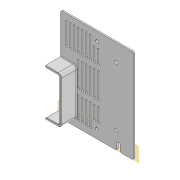
# Autodesk Inventor part: fechamento2
Saved by Autodesk Inventor 2020 (Build 240168000, 168)
## iProperties
Created: 2022-08-02
Part Number: fechamento2
Material: Genérico
Document SubType Name: Modeling
Designer: gabri
Density: 1 g/cm^3
Appearance: Padrão
Author: gabri
Autodesk Inventor part; units mm, degrees
ref_plane "YZ Plane" through (0, 0, 0) normal (1, 0, 0) x (0, 1, 0)
ref_plane "XZ Plane" through (0, 0, 0) normal (0, 1, 0) x (-1, 0, 0)
ref_plane "XY Plane" through (0, 0, 0) normal (0, 0, 1) x (1, 0, 0)
ref_plane "Plano de trabalho1" through (0, 0, 0) normal (0, 0, 1) x (1, 0, 0)
sketch "Esboço1" plane through (0, 0, 0) normal (0, 0, 1) x (1, 0, 0)
  arc A0 (62, 11) -> (61, 12) centre (61, 11) ccw projected
  line L0 (61, 12) -> (49, 12) projected
  arc A1 (49, 12) -> (48, 11) centre (49, 11) ccw projected
  line L1 (48, 1) -> (48, 11) projected
  arc A2 (47, 0) -> (48, 1) centre (47, 1) ccw projected
  line L2 (11, 0) -> (47, 0) projected
  arc A3 (10, 1) -> (11, 0) centre (11, 1) ccw projected
  line L3 (10, 1) -> (10, 9) projected
  line L4 (0, 9) -> (10, 9) projected
  line L5 (0, -8) -> (0, 9) projected
  line L6 (0, -8) -> (110, -8) projected
  line L7 (110, -8) -> (110, 9) projected
  line L8 (100, 9) -> (110, 9) projected
  line L9 (100, 1) -> (100, 9) projected
  arc A4 (99, 0) -> (100, 1) centre (99, 1) ccw projected
  line L10 (63, 0) -> (99, 0) projected
  arc A5 (62, 1) -> (63, 0) centre (63, 1) ccw projected
  line L11 (62, 11) -> (62, 1) projected
  circle A6 centre (55, 6) radius 2.25 projected
  arc A7 (48, 96) -> (49, 95) centre (49, 96) ccw projected
  line L12 (61, 95) -> (49, 95) projected
  arc A8 (61, 95) -> (62, 96) centre (61, 96) ccw projected
  line L13 (62, 106) -> (62, 96) projected
  arc A9 (63, 107) -> (62, 106) centre (63, 106) ccw projected
  line L14 (63, 107) -> (99.2679, 107) projected
  spline S0 degree 3 poles (101, 106) (100.7229, 106.2771) (100.3848, 106.6039) (99.8153, 106.9104) (99.5228, 107) (99.2679, 107) knots 0 0 0 0 0.117563 0.117563 0.194026 0.194026 0.194026 0.194026 projected
  line L15 (101, 98) -> (101, 106) projected
  line L16 (110, 98) -> (101, 98) projected
  line L17 (110, 115) -> (110, 98) projected
  line L18 (0, 115) -> (110, 115) projected
  line L19 (0, 115) -> (0, 98) projected
  line L20 (10, 98) -> (0, 98) projected
  line L21 (10, 106) -> (10, 98) projected
  arc A10 (11, 107) -> (10, 106) centre (11, 106) ccw projected
  line L22 (11, 107) -> (47, 107) projected
  arc A11 (48, 106) -> (47, 107) centre (47, 106) ccw projected
  line L23 (48, 96) -> (48, 106) projected
  circle A12 centre (55, 101) radius 2.25 projected
  line L24 (109.5, 114) -> (0.5, 114)
  line L25 (0.5, 114) -> (0.5, -7)
  line L26 (0.5, -7) -> (109.5, -7)
  line L27 (109.5, -7) -> (109.5, 114)
  line L28 (55, 101.5) -> (55, 100.5)
  line L29 (55, 101.5) -> (55, 100.5) construction
  line L30 (52.75, 101.5) -> (52.75, 100.5)
  line L31 (57.25, 100.5) -> (57.25, 101.5)
  arc A13 (57.25, 101.5) -> (52.75, 101.5) centre (55, 101.5) ccw
  arc A14 (52.75, 100.5) -> (57.25, 100.5) centre (55, 100.5) ccw
  circle A15 centre (55, 6) radius 0.25
  line L32 (55, 6.25) -> (55, 5.75) construction
  line L33 (52.75, 6.25) -> (52.75, 5.75)
  line L34 (57.25, 5.75) -> (57.25, 6.25)
  arc A16 (57.25, 6.25) -> (52.75, 6.25) centre (55, 6.25) ccw
  arc A17 (52.75, 5.75) -> (57.25, 5.75) centre (55, 5.75) ccw
  circle A18 centre (86.5, 96) radius 5
  circle A19 centre (86.5, 65) radius 5
  line L35 (45.1388, 99) -> (45.1388, 67) construction
  line L36 (46.7388, 99) -> (46.7388, 67)
  line L37 (43.5388, 67) -> (43.5388, 99)
  arc A20 (46.7388, 99) -> (43.5388, 99) centre (45.1388, 99) ccw
  arc A21 (43.5388, 67) -> (46.7388, 67) centre (45.1388, 67) ccw
  line L38 (45.1388, 35) -> (45.1388, 3) construction
  line L39 (46.7388, 35) -> (46.7388, 3)
  line L40 (43.5388, 3) -> (43.5388, 35)
  arc A22 (46.7388, 35) -> (43.5388, 35) centre (45.1388, 35) ccw
  arc A23 (43.5388, 3) -> (46.7388, 3) centre (45.1388, 3) ccw
  arc A24 (37.5388, 67) -> (40.7388, 67) centre (39.1388, 67) ccw
  arc A25 (40.7388, 35) -> (37.5388, 35) centre (39.1388, 35) ccw
  line L41 (40.7388, 99) -> (40.7388, 67)
  line L42 (39.1388, 99) -> (39.1388, 67) construction
  line L43 (37.5388, 67) -> (37.5388, 99)
  arc A26 (40.7388, 99) -> (37.5388, 99) centre (39.1388, 99) ccw
  line L44 (40.7388, 35) -> (40.7388, 3)
  line L45 (39.1388, 35) -> (39.1388, 3) construction
  line L46 (37.5388, 3) -> (37.5388, 35)
  arc A27 (37.5388, 3) -> (40.7388, 3) centre (39.1388, 3) ccw
  arc A28 (31.5388, 67) -> (34.7388, 67) centre (33.1388, 67) ccw
  arc A29 (34.7388, 35) -> (31.5388, 35) centre (33.1388, 35) ccw
  line L47 (34.7388, 99) -> (34.7388, 67)
  line L48 (33.1388, 99) -> (33.1388, 67) construction
  line L49 (31.5388, 67) -> (31.5388, 99)
  arc A30 (34.7388, 99) -> (31.5388, 99) centre (33.1388, 99) ccw
  line L50 (34.7388, 35) -> (34.7388, 3)
  line L51 (33.1388, 35) -> (33.1388, 3) construction
  line L52 (31.5388, 3) -> (31.5388, 35)
  arc A31 (31.5388, 3) -> (34.7388, 3) centre (33.1388, 3) ccw
  arc A32 (25.5388, 67) -> (28.7388, 67) centre (27.1388, 67) ccw
  arc A33 (28.7388, 35) -> (25.5388, 35) centre (27.1388, 35) ccw
  line L53 (28.7388, 99) -> (28.7388, 67)
  line L54 (27.1388, 99) -> (27.1388, 67) construction
  line L55 (25.5388, 67) -> (25.5388, 99)
  arc A34 (28.7388, 99) -> (25.5388, 99) centre (27.1388, 99) ccw
  line L56 (28.7388, 35) -> (28.7388, 3)
  line L57 (27.1388, 35) -> (27.1388, 3) construction
  line L58 (25.5388, 3) -> (25.5388, 35)
  arc A35 (25.5388, 3) -> (28.7388, 3) centre (27.1388, 3) ccw
  arc A36 (19.5388, 67) -> (22.7388, 67) centre (21.1388, 67) ccw
  arc A37 (22.7388, 35) -> (19.5388, 35) centre (21.1388, 35) ccw
  line L59 (22.7388, 99) -> (22.7388, 67)
  line L60 (21.1388, 99) -> (21.1388, 67) construction
  line L61 (19.5388, 67) -> (19.5388, 99)
  arc A38 (22.7388, 99) -> (19.5388, 99) centre (21.1388, 99) ccw
  line L62 (22.7388, 35) -> (22.7388, 3)
  line L63 (21.1388, 35) -> (21.1388, 3) construction
  line L64 (19.5388, 3) -> (19.5388, 35)
  arc A39 (19.5388, 3) -> (22.7388, 3) centre (21.1388, 3) ccw
  arc A40 (13.5388, 67) -> (16.7388, 67) centre (15.1388, 67) ccw
  arc A41 (16.7388, 35) -> (13.5388, 35) centre (15.1388, 35) ccw
  line L65 (16.7388, 99) -> (16.7388, 67)
  line L66 (15.1388, 99) -> (15.1388, 67) construction
  line L67 (13.5388, 67) -> (13.5388, 99)
  arc A42 (16.7388, 99) -> (13.5388, 99) centre (15.1388, 99) ccw
  line L68 (16.7388, 35) -> (16.7388, 3)
  line L69 (15.1388, 35) -> (15.1388, 3) construction
  line L70 (13.5388, 3) -> (13.5388, 35)
  arc A43 (13.5388, 3) -> (16.7388, 3) centre (15.1388, 3) ccw
  arc A44 (7.5388, 67) -> (10.7388, 67) centre (9.1388, 67) ccw
  arc A45 (10.7388, 35) -> (7.5388, 35) centre (9.1388, 35) ccw
  line L71 (10.7388, 99) -> (10.7388, 67)
  line L72 (9.1388, 99) -> (9.1388, 67) construction
  line L73 (7.5388, 67) -> (7.5388, 99)
  arc A46 (10.7388, 99) -> (7.5388, 99) centre (9.1388, 99) ccw
  line L74 (10.7388, 35) -> (10.7388, 3)
  line L75 (9.1388, 35) -> (9.1388, 3) construction
  line L76 (7.5388, 3) -> (7.5388, 35)
  arc A47 (7.5388, 3) -> (10.7388, 3) centre (9.1388, 3) ccw
  line L77 (51.1388, 35) -> (51.1388, 15.5537) construction
  line L78 (49.5388, 35) -> (49.5388, 15.5537)
  line L79 (52.7388, 15.5537) -> (52.7388, 35)
  arc A48 (52.7388, 35) -> (49.5388, 35) centre (51.1388, 35) ccw
  arc A49 (49.5388, 15.5537) -> (52.7388, 15.5537) centre (51.1388, 15.5537) ccw
  line L80 (55.5388, 35) -> (55.5388, 15.5537)
  line L81 (57.1388, 35) -> (57.1388, 15.5537) construction
  arc A50 (55.5388, 15.5537) -> (58.7388, 15.5537) centre (57.1388, 15.5537) ccw
  line L82 (58.7388, 15.5537) -> (58.7388, 35)
  arc A51 (58.7388, 35) -> (55.5388, 35) centre (57.1388, 35) ccw
  line L83 (61.5388, 35) -> (61.5388, 15.5537)
  line L84 (63.1388, 35) -> (63.1388, 15.5537) construction
  arc A52 (61.5388, 15.5537) -> (64.7388, 15.5537) centre (63.1388, 15.5537) ccw
  line L85 (64.7388, 15.5537) -> (64.7388, 35)
  arc A53 (64.7388, 35) -> (61.5388, 35) centre (63.1388, 35) ccw
  line L86 (69.1388, 35) -> (69.1388, 3) construction
  line L87 (67.5388, 35) -> (67.5388, 3)
  line L88 (70.7388, 3) -> (70.7388, 35)
  arc A54 (70.7388, 35) -> (67.5388, 35) centre (69.1388, 35) ccw
  arc A55 (67.5388, 3) -> (70.7388, 3) centre (69.1388, 3) ccw
  arc A56 (76.7388, 35) -> (73.5388, 35) centre (75.1388, 35) ccw
  line L89 (73.5388, 35) -> (73.5388, 3)
  line L90 (75.1388, 35) -> (75.1388, 3) construction
  arc A57 (73.5388, 3) -> (76.7388, 3) centre (75.1388, 3) ccw
  line L91 (76.7388, 3) -> (76.7388, 35)
  arc A58 (82.7388, 35) -> (79.5388, 35) centre (81.1388, 35) ccw
  line L92 (79.5388, 35) -> (79.5388, 3)
  line L93 (81.1388, 35) -> (81.1388, 3) construction
  arc A59 (79.5388, 3) -> (82.7388, 3) centre (81.1388, 3) ccw
  line L94 (82.7388, 3) -> (82.7388, 35)
  arc A60 (88.7388, 35) -> (85.5388, 35) centre (87.1388, 35) ccw
  line L95 (85.5388, 35) -> (85.5388, 3)
  line L96 (87.1388, 35) -> (87.1388, 3) construction
  arc A61 (85.5388, 3) -> (88.7388, 3) centre (87.1388, 3) ccw
  line L97 (88.7388, 3) -> (88.7388, 35)
  arc A62 (94.7388, 35) -> (91.5388, 35) centre (93.1388, 35) ccw
  line L98 (91.5388, 35) -> (91.5388, 3)
  line L99 (93.1388, 35) -> (93.1388, 3) construction
  arc A63 (91.5388, 3) -> (94.7388, 3) centre (93.1388, 3) ccw
  line L100 (94.7388, 3) -> (94.7388, 35)
  line L101 (97.5388, 35) -> (97.5388, 3)
  line L102 (99.1388, 35) -> (99.1388, 3) construction
  line L103 (100.7388, 3) -> (100.7388, 35)
  arc A64 (100.7388, 35) -> (97.5388, 35) centre (99.1388, 35) ccw
  arc A65 (97.5388, 3) -> (100.7388, 3) centre (99.1388, 3) ccw
  point P0 (0, 0)
  point P1 (55, 101)
  point P2 (45.1388, 83)
  point P3 (45.1388, 19)
  point P4 (42, 106)
  point P5 (39.1388, 83)
  point P6 (39.1388, 19)
  point P7 (36, 106)
  point P8 (33.1388, 83)
  point P9 (33.1388, 19)
  point P10 (30, 106)
  point P11 (27.1388, 83)
  point P12 (27.1388, 19)
  point P13 (24, 106)
  point P14 (21.1388, 83)
  point P15 (21.1388, 19)
  point P16 (18, 106)
  point P17 (15.1388, 83)
  point P18 (15.1388, 19)
  point P19 (12, 106)
  point P20 (9.1388, 83)
  point P21 (9.1388, 19)
  point P22 (51.1388, 25.2768)
  point P23 (57.1388, 25.2768)
  point P24 (63.1388, 25.2768)
  point P25 (69.1388, 19)
  point P26 (75.1388, 19)
  point P27 (81.1388, 19)
  point P28 (87.1388, 19)
  point P29 (93.1388, 19)
  point P30 (99.1388, 19)
  point P31 (10, 100.3484)
  point P32 (7.5388, 98)
  dimension "d0" = 0.5
  dimension "d1" = 0.5
  dimension "d2" = 1
  dimension "d3" = 1
  dimension "d4" = 0.5
  dimension "d5" = 0.5
  dimension "d6" = 4.5
  dimension "d7" = 0.5
  dimension "d8" = 4.5
  dimension "d9" = 10
  dimension "d10" = 10
  dimension "d11" = 18
  dimension "d12" = 23
  dimension "d13" = 23
  dimension "d14" = 31
  dimension "d15" = 32
  dimension "d16" = 32
  dimension "d17" = 31
  dimension "d18" = 26
  dimension "d19" = 3.2
  dimension "d20" = 3.2
  dimension "d23" = 6
  dimension "d30" = 3.2
  dimension "d31" = 6
  dimension "d34" = 6
  dimension "d39" = 3.2
  dimension "d40" = 6
  dimension "d43" = 6
  dimension "d50" = 6
  dimension "d69" = 32
  dimension "d70" = 26
  dimension "d71" = 19.4463
  dimension "d72" = 32.2769
  constraints: 210 end point, 102 point on circle, 53 centre point, 24 tangent, 14 point on line, 9 equal length, 6 midpoint, 5 horizontal, 5 vertical, 1 coincident, 1 perpendicular, 234 other
  measures "d0" distance between parallel lines of L17 L27
  measures "d1" distance from line of L19.end L25
  measures "d2" distance between parallel lines of L18 L24
  measures "d3" distance between parallel lines of L6 L26
  measures "d4" distance of L28.start A12.centre
  measures "d5" distance of L28.end A12.centre
  measures "d6" diameter of A14
  measures "d7" diameter of A15
  measures "d8" diameter of A17
  measures "d9" diameter of A18
  measures "d10" diameter of A19
  measures "d11" distance from line of L24 A18.centre
  measures "d12" distance from line of L27 A18.centre
  measures "d13" distance from line of L27 A19.centre
  measures "d14" distance of A19.centre A18.centre
  measures "d15" distance of L35.start L35.end
  measures "d16" distance of L38.start L38.end
  measures "d17" distance from line of L24 point (45.139, 83)
  measures "d18" distance from line of L26 point (45.139, 19)
  measures "d19" distance between parallel lines of L37 L36
  measures "d20" distance between parallel lines of L40 L39
  measures "d23" distance of L23.end point (42, 106)
  measures "d30" diameter of A49
  measures "d31" distance between parallel lines of L40 L78
  measures "d34" distance of L77.start L81.start
  measures "d39" diameter of A55
  measures "d40" horizontal distance of point (63.139, 25.277) point (69.139, 19)
  measures "d43" distance of L86.start L90.start
  measures "d50" distance of L98.start L101.start
  measures "d69" distance of L103.start L103.end
  measures "d70" distance from line of L26 point (69.139, 19)
  measures "d71" distance of L85.start L85.end
  measures "d72" distance from line of L26 point (57.139, 25.277)
extrude "Extrusão1" add sketch "Esboço1" along normal blind 2 contours L11 A5 L10 A4 L9 A65 L103 L8 L27 L26 L25 L4 L76 A47 L3 A3 L2 A2 L1 A1 L0 A0 | A0 L0 A1 L1 A2 L2 A3 L3 A47 L74 A45 L76 L4 L25 L20 L73 A44 L71 A46 L21 A10 L22 A11 L23 A7 L12 A8 L13 A9 L14 S0 L15 L16 L27 L8 L103 A64 L101 A65 L9 A4 L10 A5 L11 | L16 L15 S0 L14 A9 L13 A8 L12 A7 L23 A11 L22 A10 L21 A46 L73 L20 L25 L24 L27 | L20 L21 A46 L71 A44 L73 | A19 | L36 A21 L37 A20 | L43 A26 L41 A24 | L49 A30 L47 A28 | L55 A34 L53 A32 | L61 A38 L59 A36 | L67 A42 L65 A40
fillet "Arredondamento2" radius 2 4 edges at (109.5, -7, 1) (0.5, -7, 1) (0.5, 114, 1) (109.5, 114, 1)
sketch "Esboço5" plane through (0, 0, 2) normal (0, 0, 1) x (1, 0, 0)
  line L0 (115.4408, 125.4617) -> (-12.5595, 125.4617)
  line L1 (-12.5595, 125.4617) -> (-12.5595, 63)
  line L2 (-12.5595, 63) -> (115.4408, 63)
  line L3 (115.4408, 63) -> (115.4408, 125.4617)
  line L4 (2.5, -7) -> (107.5, -7) projected
  point P0 (0, 0)
  dimension "d66" = 70
  constraints: 8 end point, 2 parallel, 1 horizontal, 1 perpendicular
  measures "d66" distance between parallel lines of L4 L2
extrude "Extrusão5" cut sketch "Esboço5" against normal blind 2.2
mirror "Espelhamento1" about plane through (115.4408, 63, 2) normal (0, 1, 0)
sketch "Esboço6" plane through (0, 0, 2) normal (0, 0, 1) x (1, 0, 0)
  line L0 (0.5, 131) -> (0.5, -5) projected
  line L1 (0.5, 63) -> (46.0074, 63)
  arc A0 (7.5388, 91) -> (10.7388, 91) centre (9.1388, 91) ccw projected
  line L2 (9.1388, 89.4) -> (9.1388, 36.6)
  arc A1 (10.7388, 35) -> (7.5388, 35) centre (9.1388, 35) ccw projected
  line L3 (9.1388, 44.7338) -> (9.1388, 81.2662) construction
  line L4 (10.7388, 44.7338) -> (10.7388, 81.2662)
  line L5 (7.5388, 81.2662) -> (7.5388, 44.7338)
  arc A2 (7.5388, 44.7338) -> (10.7388, 44.7338) centre (9.1388, 44.7338) ccw
  arc A3 (10.7388, 81.2662) -> (7.5388, 81.2662) centre (9.1388, 81.2662) ccw
  line L6 (15.1388, 44.7338) -> (15.1388, 81.2662) construction
  line L7 (16.7388, 44.7338) -> (16.7388, 81.2662)
  line L8 (13.5388, 81.2662) -> (13.5388, 44.7338)
  arc A4 (13.5388, 44.7338) -> (16.7388, 44.7338) centre (15.1388, 44.7338) ccw
  arc A5 (16.7388, 81.2662) -> (13.5388, 81.2662) centre (15.1388, 81.2662) ccw
  line L9 (21.1388, 44.7338) -> (21.1388, 81.2662) construction
  line L10 (22.7388, 44.7338) -> (22.7388, 81.2662)
  line L11 (19.5388, 81.2662) -> (19.5388, 44.7338)
  arc A6 (19.5388, 44.7338) -> (22.7388, 44.7338) centre (21.1388, 44.7338) ccw
  arc A7 (22.7388, 81.2662) -> (19.5388, 81.2662) centre (21.1388, 81.2662) ccw
  line L12 (27.1388, 44.7338) -> (27.1388, 81.2662) construction
  line L13 (28.7388, 44.7338) -> (28.7388, 81.2662)
  line L14 (25.5388, 81.2662) -> (25.5388, 44.7338)
  arc A8 (25.5388, 44.7338) -> (28.7388, 44.7338) centre (27.1388, 44.7338) ccw
  arc A9 (28.7388, 81.2662) -> (25.5388, 81.2662) centre (27.1388, 81.2662) ccw
  line L15 (33.1388, 44.7338) -> (33.1388, 81.2662) construction
  line L16 (34.7388, 44.7338) -> (34.7388, 81.2662)
  line L17 (31.5388, 81.2662) -> (31.5388, 44.7338)
  arc A10 (31.5388, 44.7338) -> (34.7388, 44.7338) centre (33.1388, 44.7338) ccw
  arc A11 (34.7388, 81.2662) -> (31.5388, 81.2662) centre (33.1388, 81.2662) ccw
  line L18 (39.1388, 44.7338) -> (39.1388, 81.2662) construction
  line L19 (40.7388, 44.7338) -> (40.7388, 81.2662)
  line L20 (37.5388, 81.2662) -> (37.5388, 44.7338)
  arc A12 (37.5388, 44.7338) -> (40.7388, 44.7338) centre (39.1388, 44.7338) ccw
  arc A13 (40.7388, 81.2662) -> (37.5388, 81.2662) centre (39.1388, 81.2662) ccw
  line L21 (45.1388, 44.7338) -> (45.1388, 81.2662) construction
  line L22 (46.7388, 44.7338) -> (46.7388, 81.2662)
  line L23 (43.5388, 81.2662) -> (43.5388, 44.7338)
  arc A14 (43.5388, 44.7338) -> (46.7388, 44.7338) centre (45.1388, 44.7338) ccw
  arc A15 (46.7388, 81.2662) -> (43.5388, 81.2662) centre (45.1388, 81.2662) ccw
  line L24 (51.1388, 44.7338) -> (51.1388, 81.2662) construction
  line L25 (52.7388, 44.7338) -> (52.7388, 81.2662)
  line L26 (49.5388, 81.2662) -> (49.5388, 44.7338)
  arc A16 (49.5388, 44.7338) -> (52.7388, 44.7338) centre (51.1388, 44.7338) ccw
  arc A17 (52.7388, 81.2662) -> (49.5388, 81.2662) centre (51.1388, 81.2662) ccw
  line L27 (57.1388, 44.7338) -> (57.1388, 81.2662) construction
  line L28 (58.7388, 44.7338) -> (58.7388, 81.2662)
  line L29 (55.5388, 81.2662) -> (55.5388, 44.7338)
  arc A18 (55.5388, 44.7338) -> (58.7388, 44.7338) centre (57.1388, 44.7338) ccw
  arc A19 (58.7388, 81.2662) -> (55.5388, 81.2662) centre (57.1388, 81.2662) ccw
  line L30 (63.1388, 44.7338) -> (63.1388, 81.2662) construction
  line L31 (64.7388, 44.7338) -> (64.7388, 81.2662)
  line L32 (61.5388, 81.2662) -> (61.5388, 44.7338)
  arc A20 (61.5388, 44.7338) -> (64.7388, 44.7338) centre (63.1388, 44.7338) ccw
  arc A21 (64.7388, 81.2662) -> (61.5388, 81.2662) centre (63.1388, 81.2662) ccw
  line L33 (69.1388, 44.7338) -> (69.1388, 81.2662) construction
  line L34 (70.7388, 44.7338) -> (70.7388, 81.2662)
  line L35 (67.5388, 81.2662) -> (67.5388, 44.7338)
  arc A22 (67.5388, 44.7338) -> (70.7388, 44.7338) centre (69.1388, 44.7338) ccw
  arc A23 (70.7388, 81.2662) -> (67.5388, 81.2662) centre (69.1388, 81.2662) ccw
  point P0 (0, 0)
  point P1 (9.1388, 63)
  point P2 (15.1388, 63)
  point P3 (21.1388, 63)
  point P4 (27.1388, 63)
  point P5 (33.1388, 63)
  point P6 (39.1388, 63)
  point P7 (45.1388, 63)
  point P8 (51.1388, 63)
  point P9 (57.1388, 63)
  point P10 (63.1388, 63)
  point P11 (69.1388, 63)
  dimension "d73" = 3.2
  dimension "d76" = 6
  constraints: 92 end point, 46 point on circle, 22 centre point, 4 tangent, 3 midpoint, 2 horizontal, 1 parallel, 1 point on line, 1 vertical, 120 other
  measures "d73" distance between parallel lines of L5 L4
  measures "d76" distance of L4.start L7.start
extrude "Extrusão6" cut sketch "Esboço6" against normal blind 2.2
sketch "Esboço7" plane through (0, 0, 2) normal (0, 0, 1) x (1, 0, 0)
  line L0 (21.5, -37.6747) -> (-7.1318, -37.6747)
  line L1 (-7.1318, -37.6747) -> (-7.1318, 70)
  line L2 (-7.1318, 70) -> (21.5, 70)
  line L3 (21.5, 70) -> (21.5, -37.6747)
  line L4 (2.5, -7) -> (107.5, -7) projected
  line L5 (0.5, 131) -> (0.5, -5) projected
  point P0 (0, 0)
  dimension "d83" = 77
  dimension "d84" = 21
  constraints: 8 end point, 2 parallel, 1 horizontal, 1 perpendicular
  measures "d83" distance between parallel lines of L4 L2
  measures "d84" distance between parallel lines of L3 L5
sketch "Esboço8" plane through (0, 0, 2) normal (0, 0, 1) x (1, 0, 0)
  arc A0 (19.5388, 44.7338) -> (22.7388, 44.7338) centre (21.1388, 44.7338) ccw projected
  line L0 (19.5388, 44.7338) -> (19.5388, 81.2662) projected
  arc A1 (22.7388, 81.2662) -> (19.5388, 81.2662) centre (21.1388, 81.2662) ccw projected
  line L1 (22.7388, 81.2662) -> (22.7388, 44.7338) projected
  arc A2 (43.5388, 44.7338) -> (46.7388, 44.7338) centre (45.1388, 44.7338) ccw projected
  line L2 (43.5388, 44.7338) -> (43.5388, 81.2662) projected
  arc A3 (46.7388, 81.2662) -> (43.5388, 81.2662) centre (45.1388, 81.2662) ccw projected
  line L3 (46.7388, 81.2662) -> (46.7388, 44.7338) projected
  arc A4 (67.5388, 44.7338) -> (70.7388, 44.7338) centre (69.1388, 44.7338) ccw projected
  line L4 (67.5388, 44.7338) -> (67.5388, 81.2662) projected
  arc A5 (70.7388, 81.2662) -> (67.5388, 81.2662) centre (69.1388, 81.2662) ccw projected
  line L5 (70.7388, 81.2662) -> (70.7388, 44.7338) projected
  line L6 (52.7388, 81.2662) -> (52.7388, 44.7338) projected
  arc A6 (49.5388, 44.7338) -> (52.7388, 44.7338) centre (51.1388, 44.7338) ccw projected
  line L7 (49.5388, 44.7338) -> (49.5388, 81.2662) projected
  arc A7 (52.7388, 81.2662) -> (49.5388, 81.2662) centre (51.1388, 81.2662) ccw projected
  arc A8 (25.5388, 44.7338) -> (28.7388, 44.7338) centre (27.1388, 44.7338) ccw projected
  line L8 (25.5388, 44.7338) -> (25.5388, 81.2662) projected
  arc A9 (28.7388, 81.2662) -> (25.5388, 81.2662) centre (27.1388, 81.2662) ccw projected
  line L9 (28.7388, 81.2662) -> (28.7388, 44.7338) projected
  arc A10 (13.5388, 44.7338) -> (16.7388, 44.7338) centre (15.1388, 44.7338) ccw projected
  line L10 (13.5388, 44.7338) -> (13.5388, 81.2662) projected
  arc A11 (16.7388, 81.2662) -> (13.5388, 81.2662) centre (15.1388, 81.2662) ccw projected
  line L11 (16.7388, 81.2662) -> (16.7388, 44.7338) projected
  arc A12 (40.7388, 81.2662) -> (37.5388, 81.2662) centre (39.1388, 81.2662) ccw projected
  line L12 (40.7388, 81.2662) -> (40.7388, 44.7338) projected
  arc A13 (37.5388, 44.7338) -> (40.7388, 44.7338) centre (39.1388, 44.7338) ccw projected
  line L13 (37.5388, 44.7338) -> (37.5388, 81.2662) projected
  arc A14 (61.5388, 44.7338) -> (64.7388, 44.7338) centre (63.1388, 44.7338) ccw projected
  line L14 (61.5388, 44.7338) -> (61.5388, 81.2662) projected
  arc A15 (64.7388, 81.2662) -> (61.5388, 81.2662) centre (63.1388, 81.2662) ccw projected
  line L15 (64.7388, 81.2662) -> (64.7388, 44.7338) projected
  line L16 (58.7388, 81.2662) -> (58.7388, 44.7338) projected
  arc A16 (55.5388, 44.7338) -> (58.7388, 44.7338) centre (57.1388, 44.7338) ccw projected
  line L17 (55.5388, 44.7338) -> (55.5388, 81.2662) projected
  arc A17 (58.7388, 81.2662) -> (55.5388, 81.2662) centre (57.1388, 81.2662) ccw projected
  line L18 (31.5388, 44.7338) -> (31.5388, 81.2662) projected
  arc A18 (34.7388, 81.2662) -> (31.5388, 81.2662) centre (33.1388, 81.2662) ccw projected
  line L19 (34.7388, 81.2662) -> (34.7388, 44.7338) projected
  arc A19 (31.5388, 44.7338) -> (34.7388, 44.7338) centre (33.1388, 44.7338) ccw projected
  line L20 (10.7388, 81.2662) -> (10.7388, 44.7338) projected
  arc A20 (7.5388, 44.7338) -> (10.7388, 44.7338) centre (9.1388, 44.7338) ccw projected
  line L21 (7.5388, 44.7338) -> (7.5388, 81.2662) projected
  arc A21 (10.7388, 81.2662) -> (7.5388, 81.2662) centre (9.1388, 81.2662) ccw projected
  arc A22 (46.7388, 123) -> (43.5388, 123) centre (45.1388, 123) ccw projected
  line L22 (46.7388, 91) -> (46.7388, 123) projected
  arc A23 (43.5388, 91) -> (46.7388, 91) centre (45.1388, 91) ccw projected
  line L23 (43.5388, 123) -> (43.5388, 91) projected
  line L24 (19.5388, 123) -> (19.5388, 91) projected
  arc A24 (22.7388, 123) -> (19.5388, 123) centre (21.1388, 123) ccw projected
  line L25 (22.7388, 91) -> (22.7388, 123) projected
  arc A25 (19.5388, 91) -> (22.7388, 91) centre (21.1388, 91) ccw projected
  arc A26 (25.5388, 91) -> (28.7388, 91) centre (27.1388, 91) ccw projected
  line L26 (25.5388, 123) -> (25.5388, 91) projected
  arc A27 (28.7388, 123) -> (25.5388, 123) centre (27.1388, 123) ccw projected
  line L27 (28.7388, 91) -> (28.7388, 123) projected
  arc A28 (31.5388, 91) -> (34.7388, 91) centre (33.1388, 91) ccw projected
  line L28 (31.5388, 123) -> (31.5388, 91) projected
  arc A29 (34.7388, 123) -> (31.5388, 123) centre (33.1388, 123) ccw projected
  line L29 (34.7388, 91) -> (34.7388, 123) projected
  line L30 (40.7388, 91) -> (40.7388, 123) projected
  arc A30 (37.5388, 91) -> (40.7388, 91) centre (39.1388, 91) ccw projected
  line L31 (37.5388, 123) -> (37.5388, 91) projected
  arc A31 (40.7388, 123) -> (37.5388, 123) centre (39.1388, 123) ccw projected
  line L32 (49.5388, 110.4463) -> (49.5388, 91) projected
  arc A32 (52.7388, 110.4463) -> (49.5388, 110.4463) centre (51.1388, 110.4463) ccw projected
  line L33 (52.7388, 91) -> (52.7388, 110.4463) projected
  arc A33 (49.5388, 91) -> (52.7388, 91) centre (51.1388, 91) ccw projected
  arc A34 (13.5388, 91) -> (16.7388, 91) centre (15.1388, 91) ccw projected
  line L34 (13.5388, 123) -> (13.5388, 91) projected
  arc A35 (16.7388, 123) -> (13.5388, 123) centre (15.1388, 123) ccw projected
  line L35 (16.7388, 91) -> (16.7388, 123) projected
  line L36 (79.5388, 123) -> (79.5388, 91) projected
  arc A36 (82.7388, 123) -> (79.5388, 123) centre (81.1388, 123) ccw projected
  line L37 (82.7388, 91) -> (82.7388, 123) projected
  arc A37 (79.5388, 91) -> (82.7388, 91) centre (81.1388, 91) ccw projected
  line L38 (64.7388, 91) -> (64.7388, 110.4463) projected
  arc A38 (61.5388, 91) -> (64.7388, 91) centre (63.1388, 91) ccw projected
  line L39 (61.5388, 110.4463) -> (61.5388, 91) projected
  arc A39 (64.7388, 110.4463) -> (61.5388, 110.4463) centre (63.1388, 110.4463) ccw projected
  line L40 (67.5388, 123) -> (67.5388, 91) projected
  arc A40 (70.7388, 123) -> (67.5388, 123) centre (69.1388, 123) ccw projected
  line L41 (70.7388, 91) -> (70.7388, 123) projected
  arc A41 (67.5388, 91) -> (70.7388, 91) centre (69.1388, 91) ccw projected
  line L42 (73.5388, 123) -> (73.5388, 91) projected
  arc A42 (76.7388, 123) -> (73.5388, 123) centre (75.1388, 123) ccw projected
  line L43 (76.7388, 91) -> (76.7388, 123) projected
  arc A43 (73.5388, 91) -> (76.7388, 91) centre (75.1388, 91) ccw projected
  arc A44 (55.5388, 91) -> (58.7388, 91) centre (57.1388, 91) ccw projected
  line L44 (55.5388, 110.4463) -> (55.5388, 91) projected
  arc A45 (58.7388, 110.4463) -> (55.5388, 110.4463) centre (57.1388, 110.4463) ccw projected
  line L45 (58.7388, 91) -> (58.7388, 110.4463) projected
  arc A46 (88.7388, 123) -> (85.5388, 123) centre (87.1388, 123) ccw projected
  line L46 (88.7388, 91) -> (88.7388, 123) projected
  arc A47 (85.5388, 91) -> (88.7388, 91) centre (87.1388, 91) ccw projected
  line L47 (85.5388, 123) -> (85.5388, 91) projected
  line L48 (94.7388, 91) -> (94.7388, 123) projected
  arc A48 (91.5388, 91) -> (94.7388, 91) centre (93.1388, 91) ccw projected
  line L49 (91.5388, 123) -> (91.5388, 91) projected
  arc A49 (94.7388, 123) -> (91.5388, 123) centre (93.1388, 123) ccw projected
  arc A50 (57.25, 120.25) -> (52.75, 120.25) centre (55, 120.25) ccw projected
  line L50 (57.25, 119.75) -> (57.25, 120.25) projected
  arc A51 (52.75, 119.75) -> (57.25, 119.75) centre (55, 119.75) ccw projected
  line L51 (52.75, 120.25) -> (52.75, 119.75) projected
  arc A52 (7.5388, 91) -> (10.7388, 91) centre (9.1388, 91) ccw projected
  line L52 (7.5388, 123) -> (7.5388, 91) projected
  arc A53 (10.7388, 123) -> (7.5388, 123) centre (9.1388, 123) ccw projected
  line L53 (10.7388, 91) -> (10.7388, 123) projected
  arc A54 (97.5388, 91) -> (100.7388, 91) centre (99.1388, 91) ccw projected
  line L54 (97.5388, 123) -> (97.5388, 91) projected
  arc A55 (100.7388, 123) -> (97.5388, 123) centre (99.1388, 123) ccw projected
  line L55 (100.7388, 91) -> (100.7388, 123) projected
  line L56 (0.5, 131) -> (0.5, -5) projected
  arc A56 (0.5, -5) -> (2.5, -7) centre (2.5, -5) ccw projected
  line L57 (2.5, -7) -> (107.5, -7) projected
  arc A57 (107.5, -7) -> (109.5, -5) centre (107.5, -5) ccw projected
  line L58 (109.5, 131) -> (109.5, -5) projected
  arc A58 (109.5, 131) -> (107.5, 133) centre (107.5, 131) ccw projected
  line L59 (2.5, 133) -> (107.5, 133) projected
  arc A59 (2.5, 133) -> (0.5, 131) centre (2.5, 131) ccw projected
  arc A60 (100.7388, 35) -> (97.5388, 35) centre (99.1388, 35) ccw projected
  line L60 (100.7388, 35) -> (100.7388, 3) projected
  arc A61 (97.5388, 3) -> (100.7388, 3) centre (99.1388, 3) ccw projected
  line L61 (97.5388, 3) -> (97.5388, 35) projected
  arc A62 (10.7388, 35) -> (7.5388, 35) centre (9.1388, 35) ccw projected
  line L62 (10.7388, 35) -> (10.7388, 3) projected
  arc A63 (7.5388, 3) -> (10.7388, 3) centre (9.1388, 3) ccw projected
  line L63 (7.5388, 3) -> (7.5388, 35) projected
  arc A64 (52.75, 5.75) -> (57.25, 5.75) centre (55, 5.75) ccw projected
  line L64 (52.75, 5.75) -> (52.75, 6.25) projected
  arc A65 (57.25, 6.25) -> (52.75, 6.25) centre (55, 6.25) ccw projected
  line L65 (57.25, 6.25) -> (57.25, 5.75) projected
  line L66 (94.7388, 35) -> (94.7388, 3) projected
  arc A66 (91.5388, 3) -> (94.7388, 3) centre (93.1388, 3) ccw projected
  line L67 (91.5388, 3) -> (91.5388, 35) projected
  arc A67 (94.7388, 35) -> (91.5388, 35) centre (93.1388, 35) ccw projected
  arc A68 (85.5388, 3) -> (88.7388, 3) centre (87.1388, 3) ccw projected
  line L68 (85.5388, 3) -> (85.5388, 35) projected
  arc A69 (88.7388, 35) -> (85.5388, 35) centre (87.1388, 35) ccw projected
  line L69 (88.7388, 35) -> (88.7388, 3) projected
  arc A70 (58.7388, 35) -> (55.5388, 35) centre (57.1388, 35) ccw projected
  line L70 (58.7388, 35) -> (58.7388, 15.5537) projected
  arc A71 (55.5388, 15.5537) -> (58.7388, 15.5537) centre (57.1388, 15.5537) ccw projected
  line L71 (55.5388, 15.5537) -> (55.5388, 35) projected
  line L72 (73.5388, 3) -> (73.5388, 35) projected
  arc A72 (76.7388, 35) -> (73.5388, 35) centre (75.1388, 35) ccw projected
  line L73 (76.7388, 35) -> (76.7388, 3) projected
  arc A73 (73.5388, 3) -> (76.7388, 3) centre (75.1388, 3) ccw projected
  line L74 (67.5388, 3) -> (67.5388, 35) projected
  arc A74 (70.7388, 35) -> (67.5388, 35) centre (69.1388, 35) ccw projected
  line L75 (70.7388, 35) -> (70.7388, 3) projected
  arc A75 (67.5388, 3) -> (70.7388, 3) centre (69.1388, 3) ccw projected
  line L76 (64.7388, 35) -> (64.7388, 15.5537) projected
  arc A76 (61.5388, 15.5537) -> (64.7388, 15.5537) centre (63.1388, 15.5537) ccw projected
  line L77 (61.5388, 15.5537) -> (61.5388, 35) projected
  arc A77 (64.7388, 35) -> (61.5388, 35) centre (63.1388, 35) ccw projected
  line L78 (79.5388, 3) -> (79.5388, 35) projected
  arc A78 (82.7388, 35) -> (79.5388, 35) centre (81.1388, 35) ccw projected
  line L79 (82.7388, 35) -> (82.7388, 3) projected
  arc A79 (79.5388, 3) -> (82.7388, 3) centre (81.1388, 3) ccw projected
  arc A80 (16.7388, 35) -> (13.5388, 35) centre (15.1388, 35) ccw projected
  line L80 (16.7388, 35) -> (16.7388, 3) projected
  arc A81 (13.5388, 3) -> (16.7388, 3) centre (15.1388, 3) ccw projected
  line L81 (13.5388, 3) -> (13.5388, 35) projected
  line L82 (49.5388, 15.5537) -> (49.5388, 35) projected
  arc A82 (52.7388, 35) -> (49.5388, 35) centre (51.1388, 35) ccw projected
  line L83 (52.7388, 35) -> (52.7388, 15.5537) projected
  arc A83 (49.5388, 15.5537) -> (52.7388, 15.5537) centre (51.1388, 15.5537) ccw projected
  line L84 (40.7388, 35) -> (40.7388, 3) projected
  arc A84 (37.5388, 3) -> (40.7388, 3) centre (39.1388, 3) ccw projected
  line L85 (37.5388, 3) -> (37.5388, 35) projected
  arc A85 (40.7388, 35) -> (37.5388, 35) centre (39.1388, 35) ccw projected
  arc A86 (34.7388, 35) -> (31.5388, 35) centre (33.1388, 35) ccw projected
  line L86 (34.7388, 35) -> (34.7388, 3) projected
  arc A87 (31.5388, 3) -> (34.7388, 3) centre (33.1388, 3) ccw projected
  line L87 (31.5388, 3) -> (31.5388, 35) projected
  arc A88 (28.7388, 35) -> (25.5388, 35) centre (27.1388, 35) ccw projected
  line L88 (28.7388, 35) -> (28.7388, 3) projected
  arc A89 (25.5388, 3) -> (28.7388, 3) centre (27.1388, 3) ccw projected
  line L89 (25.5388, 3) -> (25.5388, 35) projected
  line L90 (19.5388, 3) -> (19.5388, 35) projected
  arc A90 (22.7388, 35) -> (19.5388, 35) centre (21.1388, 35) ccw projected
  line L91 (22.7388, 35) -> (22.7388, 3) projected
  arc A91 (19.5388, 3) -> (22.7388, 3) centre (21.1388, 3) ccw projected
  arc A92 (43.5388, 3) -> (46.7388, 3) centre (45.1388, 3) ccw projected
  line L92 (43.5388, 3) -> (43.5388, 35) projected
  arc A93 (46.7388, 35) -> (43.5388, 35) centre (45.1388, 35) ccw projected
  line L93 (46.7388, 35) -> (46.7388, 3) projected
  point P0 (0, 0)
extrude "Extrusão7" add sketch "Esboço8" against normal blind 2 contours L0 A1 L1 A0 | L10 A11 L11 A10 | L20 A20 L21 A21 | A59 L59 A58 L58 A57 L57 A56 L56 | L62 A63 L63 A62 | L80 A81 L81 A80 | L90 A90 L91 A91
extrude "Extrusão8" cut sketch "Esboço7" against normal blind 2
sketch "Esboço9" plane through (0, 0, 2) normal (0, 0, 1) x (1, 0, 0)
  line L0 (84.7, -25.3544) -> (89.7, -25.3544)
  line L1 (89.7, -25.3544) -> (89.7, 5)
  line L2 (89.7, 5) -> (84.7, 5)
  line L3 (84.7, 5) -> (84.7, -25.3544)
  line L4 (109.5, 131) -> (109.5, -5) projected
  line L5 (21.5, -7) -> (107.5, -7) projected
  point P0 (0, 0)
  point P1 (84.7, -7)
  point P2 (89.7, -7)
  dimension "d90" = 5
  dimension "d91" = 19.8
  dimension "d92" = 12
  constraints: 8 end point, 2 parallel, 1 horizontal, 1 perpendicular
  measures "d90" distance of L0.start L0.end
  measures "d91" distance between parallel lines of L4 L1
  measures "d92" distance between parallel lines of L5 L2
sketch "Esboço10" plane through (0, 0, 2) normal (0, 0, 1) x (1, 0, 0)
  circle A0 centre (93.1388, 11) radius 1.6053
  arc A1 (91.5388, 3) -> (94.7388, 3) centre (93.1388, 3) ccw projected
  line L0 (94.7388, 35) -> (94.7388, 3) projected
  line L1 (91.5388, 3) -> (91.5388, 35) projected
  circle A2 centre (87.1388, 11) radius 1.6
  line L2 (88.7388, 35) -> (88.7388, 3) projected
  line L3 (85.5388, 3) -> (85.5388, 35) projected
  arc A3 (85.5388, 3) -> (88.7388, 3) centre (87.1388, 3) ccw projected
  line L4 (21.5, 70) -> (21.5, -7) projected
  line L5 (21.5, -7) -> (107.5, -7) projected
  arc A4 (107.5, -7) -> (109.5, -5) centre (107.5, -5) ccw projected
  line L6 (109.5, 131) -> (109.5, -5) projected
  arc A5 (109.5, 131) -> (107.5, 133) centre (107.5, 131) ccw projected
  line L7 (2.5, 133) -> (107.5, 133) projected
  arc A6 (2.5, 133) -> (0.5, 131) centre (2.5, 131) ccw projected
  line L8 (0.5, 131) -> (0.5, 70) projected
  line L9 (0.5, 70) -> (21.5, 70) projected
  line L10 (43.5388, 44.7338) -> (43.5388, 81.2662) projected
  arc A7 (46.7388, 81.2662) -> (43.5388, 81.2662) centre (45.1388, 81.2662) ccw projected
  line L11 (46.7388, 81.2662) -> (46.7388, 44.7338) projected
  arc A8 (43.5388, 44.7338) -> (46.7388, 44.7338) centre (45.1388, 44.7338) ccw projected
  line L12 (67.5388, 44.7338) -> (67.5388, 81.2662) projected
  arc A9 (70.7388, 81.2662) -> (67.5388, 81.2662) centre (69.1388, 81.2662) ccw projected
  line L13 (70.7388, 81.2662) -> (70.7388, 44.7338) projected
  arc A10 (67.5388, 44.7338) -> (70.7388, 44.7338) centre (69.1388, 44.7338) ccw projected
  line L14 (52.7388, 81.2662) -> (52.7388, 44.7338) projected
  arc A11 (49.5388, 44.7338) -> (52.7388, 44.7338) centre (51.1388, 44.7338) ccw projected
  line L15 (49.5388, 44.7338) -> (49.5388, 81.2662) projected
  arc A12 (52.7388, 81.2662) -> (49.5388, 81.2662) centre (51.1388, 81.2662) ccw projected
  arc A13 (25.5388, 44.7338) -> (28.7388, 44.7338) centre (27.1388, 44.7338) ccw projected
  line L16 (25.5388, 44.7338) -> (25.5388, 81.2662) projected
  arc A14 (28.7388, 81.2662) -> (25.5388, 81.2662) centre (27.1388, 81.2662) ccw projected
  line L17 (28.7388, 81.2662) -> (28.7388, 44.7338) projected
  arc A15 (37.5388, 44.7338) -> (40.7388, 44.7338) centre (39.1388, 44.7338) ccw projected
  line L18 (37.5388, 44.7338) -> (37.5388, 81.2662) projected
  arc A16 (40.7388, 81.2662) -> (37.5388, 81.2662) centre (39.1388, 81.2662) ccw projected
  line L19 (40.7388, 81.2662) -> (40.7388, 44.7338) projected
  line L20 (61.5388, 44.7338) -> (61.5388, 81.2662) projected
  arc A17 (64.7388, 81.2662) -> (61.5388, 81.2662) centre (63.1388, 81.2662) ccw projected
  line L21 (64.7388, 81.2662) -> (64.7388, 44.7338) projected
  arc A18 (61.5388, 44.7338) -> (64.7388, 44.7338) centre (63.1388, 44.7338) ccw projected
  arc A19 (58.7388, 81.2662) -> (55.5388, 81.2662) centre (57.1388, 81.2662) ccw projected
  line L22 (58.7388, 81.2662) -> (58.7388, 44.7338) projected
  arc A20 (55.5388, 44.7338) -> (58.7388, 44.7338) centre (57.1388, 44.7338) ccw projected
  line L23 (55.5388, 44.7338) -> (55.5388, 81.2662) projected
  line L24 (34.7388, 81.2662) -> (34.7388, 44.7338) projected
  arc A21 (31.5388, 44.7338) -> (34.7388, 44.7338) centre (33.1388, 44.7338) ccw projected
  line L25 (31.5388, 44.7338) -> (31.5388, 81.2662) projected
  arc A22 (34.7388, 81.2662) -> (31.5388, 81.2662) centre (33.1388, 81.2662) ccw projected
  line L26 (46.7388, 91) -> (46.7388, 123) projected
  arc A23 (43.5388, 91) -> (46.7388, 91) centre (45.1388, 91) ccw projected
  line L27 (43.5388, 123) -> (43.5388, 91) projected
  arc A24 (46.7388, 123) -> (43.5388, 123) centre (45.1388, 123) ccw projected
  arc A25 (19.5388, 91) -> (22.7388, 91) centre (21.1388, 91) ccw projected
  line L28 (19.5388, 123) -> (19.5388, 91) projected
  arc A26 (22.7388, 123) -> (19.5388, 123) centre (21.1388, 123) ccw projected
  line L29 (22.7388, 91) -> (22.7388, 123) projected
  line L30 (25.5388, 123) -> (25.5388, 91) projected
  arc A27 (28.7388, 123) -> (25.5388, 123) centre (27.1388, 123) ccw projected
  line L31 (28.7388, 91) -> (28.7388, 123) projected
  arc A28 (25.5388, 91) -> (28.7388, 91) centre (27.1388, 91) ccw projected
  line L32 (31.5388, 123) -> (31.5388, 91) projected
  arc A29 (34.7388, 123) -> (31.5388, 123) centre (33.1388, 123) ccw projected
  line L33 (34.7388, 91) -> (34.7388, 123) projected
  arc A30 (31.5388, 91) -> (34.7388, 91) centre (33.1388, 91) ccw projected
  arc A31 (40.7388, 123) -> (37.5388, 123) centre (39.1388, 123) ccw projected
  line L34 (40.7388, 91) -> (40.7388, 123) projected
  arc A32 (37.5388, 91) -> (40.7388, 91) centre (39.1388, 91) ccw projected
  line L35 (37.5388, 123) -> (37.5388, 91) projected
  arc A33 (49.5388, 91) -> (52.7388, 91) centre (51.1388, 91) ccw projected
  line L36 (49.5388, 110.4463) -> (49.5388, 91) projected
  arc A34 (52.7388, 110.4463) -> (49.5388, 110.4463) centre (51.1388, 110.4463) ccw projected
  line L37 (52.7388, 91) -> (52.7388, 110.4463) projected
  line L38 (13.5388, 123) -> (13.5388, 91) projected
  arc A35 (16.7388, 123) -> (13.5388, 123) centre (15.1388, 123) ccw projected
  line L39 (16.7388, 91) -> (16.7388, 123) projected
  arc A36 (13.5388, 91) -> (16.7388, 91) centre (15.1388, 91) ccw projected
  arc A37 (79.5388, 91) -> (82.7388, 91) centre (81.1388, 91) ccw projected
  line L40 (79.5388, 123) -> (79.5388, 91) projected
  arc A38 (82.7388, 123) -> (79.5388, 123) centre (81.1388, 123) ccw projected
  line L41 (82.7388, 91) -> (82.7388, 123) projected
  arc A39 (61.5388, 91) -> (64.7388, 91) centre (63.1388, 91) ccw projected
  line L42 (61.5388, 110.4463) -> (61.5388, 91) projected
  arc A40 (64.7388, 110.4463) -> (61.5388, 110.4463) centre (63.1388, 110.4463) ccw projected
  line L43 (64.7388, 91) -> (64.7388, 110.4463) projected
  arc A41 (67.5388, 91) -> (70.7388, 91) centre (69.1388, 91) ccw projected
  line L44 (67.5388, 123) -> (67.5388, 91) projected
  arc A42 (70.7388, 123) -> (67.5388, 123) centre (69.1388, 123) ccw projected
  line L45 (70.7388, 91) -> (70.7388, 123) projected
  arc A43 (73.5388, 91) -> (76.7388, 91) centre (75.1388, 91) ccw projected
  line L46 (73.5388, 123) -> (73.5388, 91) projected
  arc A44 (76.7388, 123) -> (73.5388, 123) centre (75.1388, 123) ccw projected
  line L47 (76.7388, 91) -> (76.7388, 123) projected
  line L48 (55.5388, 110.4463) -> (55.5388, 91) projected
  arc A45 (58.7388, 110.4463) -> (55.5388, 110.4463) centre (57.1388, 110.4463) ccw projected
  line L49 (58.7388, 91) -> (58.7388, 110.4463) projected
  arc A46 (55.5388, 91) -> (58.7388, 91) centre (57.1388, 91) ccw projected
  line L50 (88.7388, 91) -> (88.7388, 123) projected
  arc A47 (85.5388, 91) -> (88.7388, 91) centre (87.1388, 91) ccw projected
  line L51 (85.5388, 123) -> (85.5388, 91) projected
  arc A48 (88.7388, 123) -> (85.5388, 123) centre (87.1388, 123) ccw projected
  arc A49 (91.5388, 91) -> (94.7388, 91) centre (93.1388, 91) ccw projected
  line L52 (91.5388, 123) -> (91.5388, 91) projected
  arc A50 (94.7388, 123) -> (91.5388, 123) centre (93.1388, 123) ccw projected
  line L53 (94.7388, 91) -> (94.7388, 123) projected
  line L54 (52.75, 120.25) -> (52.75, 119.75) projected
  arc A51 (57.25, 120.25) -> (52.75, 120.25) centre (55, 120.25) ccw projected
  line L55 (57.25, 119.75) -> (57.25, 120.25) projected
  arc A52 (52.75, 119.75) -> (57.25, 119.75) centre (55, 119.75) ccw projected
  arc A53 (7.5388, 91) -> (10.7388, 91) centre (9.1388, 91) ccw projected
  line L56 (7.5388, 123) -> (7.5388, 91) projected
  arc A54 (10.7388, 123) -> (7.5388, 123) centre (9.1388, 123) ccw projected
  line L57 (10.7388, 91) -> (10.7388, 123) projected
  line L58 (100.7388, 91) -> (100.7388, 123) projected
  arc A55 (97.5388, 91) -> (100.7388, 91) centre (99.1388, 91) ccw projected
  line L59 (97.5388, 123) -> (97.5388, 91) projected
  arc A56 (100.7388, 123) -> (97.5388, 123) centre (99.1388, 123) ccw projected
  line L60 (100.7388, 35) -> (100.7388, 3) projected
  arc A57 (97.5388, 3) -> (100.7388, 3) centre (99.1388, 3) ccw projected
  line L61 (97.5388, 3) -> (97.5388, 35) projected
  arc A58 (100.7388, 35) -> (97.5388, 35) centre (99.1388, 35) ccw projected
  line L62 (52.75, 5.75) -> (52.75, 6.25) projected
  arc A59 (57.25, 6.25) -> (52.75, 6.25) centre (55, 6.25) ccw projected
  line L63 (57.25, 6.25) -> (57.25, 5.75) projected
  arc A60 (52.75, 5.75) -> (57.25, 5.75) centre (55, 5.75) ccw projected
  arc A61 (94.7388, 35) -> (91.5388, 35) centre (93.1388, 35) ccw projected
  line L64 (94.7388, 35) -> (94.7388, 3) projected
  arc A62 (91.5388, 3) -> (94.7388, 3) centre (93.1388, 3) ccw projected
  line L65 (91.5388, 3) -> (91.5388, 35) projected
  line L66 (88.7388, 35) -> (88.7388, 3) projected
  arc A63 (85.5388, 3) -> (88.7388, 3) centre (87.1388, 3) ccw projected
  line L67 (85.5388, 3) -> (85.5388, 35) projected
  arc A64 (88.7388, 35) -> (85.5388, 35) centre (87.1388, 35) ccw projected
  line L68 (55.5388, 15.5537) -> (55.5388, 35) projected
  arc A65 (58.7388, 35) -> (55.5388, 35) centre (57.1388, 35) ccw projected
  line L69 (58.7388, 35) -> (58.7388, 15.5537) projected
  arc A66 (55.5388, 15.5537) -> (58.7388, 15.5537) centre (57.1388, 15.5537) ccw projected
  arc A67 (76.7388, 35) -> (73.5388, 35) centre (75.1388, 35) ccw projected
  line L70 (76.7388, 35) -> (76.7388, 3) projected
  arc A68 (73.5388, 3) -> (76.7388, 3) centre (75.1388, 3) ccw projected
  line L71 (73.5388, 3) -> (73.5388, 35) projected
  arc A69 (70.7388, 35) -> (67.5388, 35) centre (69.1388, 35) ccw projected
  line L72 (70.7388, 35) -> (70.7388, 3) projected
  arc A70 (67.5388, 3) -> (70.7388, 3) centre (69.1388, 3) ccw projected
  line L73 (67.5388, 3) -> (67.5388, 35) projected
  arc A71 (64.7388, 35) -> (61.5388, 35) centre (63.1388, 35) ccw projected
  line L74 (64.7388, 35) -> (64.7388, 15.5537) projected
  arc A72 (61.5388, 15.5537) -> (64.7388, 15.5537) centre (63.1388, 15.5537) ccw projected
  line L75 (61.5388, 15.5537) -> (61.5388, 35) projected
  arc A73 (82.7388, 35) -> (79.5388, 35) centre (81.1388, 35) ccw projected
  line L76 (82.7388, 35) -> (82.7388, 3) projected
  arc A74 (79.5388, 3) -> (82.7388, 3) centre (81.1388, 3) ccw projected
  line L77 (79.5388, 3) -> (79.5388, 35) projected
  arc A75 (52.7388, 35) -> (49.5388, 35) centre (51.1388, 35) ccw projected
  line L78 (52.7388, 35) -> (52.7388, 15.5537) projected
  arc A76 (49.5388, 15.5537) -> (52.7388, 15.5537) centre (51.1388, 15.5537) ccw projected
  line L79 (49.5388, 15.5537) -> (49.5388, 35) projected
  arc A77 (37.5388, 3) -> (40.7388, 3) centre (39.1388, 3) ccw projected
  line L80 (37.5388, 3) -> (37.5388, 35) projected
  arc A78 (40.7388, 35) -> (37.5388, 35) centre (39.1388, 35) ccw projected
  line L81 (40.7388, 35) -> (40.7388, 3) projected
  line L82 (31.5388, 3) -> (31.5388, 35) projected
  arc A79 (34.7388, 35) -> (31.5388, 35) centre (33.1388, 35) ccw projected
  line L83 (34.7388, 35) -> (34.7388, 3) projected
  arc A80 (31.5388, 3) -> (34.7388, 3) centre (33.1388, 3) ccw projected
  line L84 (25.5388, 3) -> (25.5388, 35) projected
  arc A81 (28.7388, 35) -> (25.5388, 35) centre (27.1388, 35) ccw projected
  line L85 (28.7388, 35) -> (28.7388, 3) projected
  arc A82 (25.5388, 3) -> (28.7388, 3) centre (27.1388, 3) ccw projected
  line L86 (46.7388, 35) -> (46.7388, 3) projected
  arc A83 (43.5388, 3) -> (46.7388, 3) centre (45.1388, 3) ccw projected
  line L87 (43.5388, 3) -> (43.5388, 35) projected
  arc A84 (46.7388, 35) -> (43.5388, 35) centre (45.1388, 35) ccw projected
  point P0 (0, 0)
  point P1 (88.7388, 11)
  point P2 (85.5388, 11)
  point P3 (91.5388, 11.1301)
  point P4 (91.5388, 10.8699)
  point P5 (94.7388, 10.8699)
  point P6 (94.7388, 11.1301)
  dimension "d93" = 8
  constraints: 2 centre point
  measures "d93" distance of A1.centre A0.centre
extrude "Extrusão9" add sketch "Esboço10" against normal blind 2 contours A0 L0 | L0 A0 L1 | A0 L1 A61 L0 | L0 A1 L1 A0 | L1 A0 | A2 | L2 A3 L3 A2 | A2 L3 A64 L2 | L12 A9 L13 A10 | L20 A17 L21 A18 | L40 A38 L41 A37 | L42 A40 L43 A39 | L44 A42 L45 A41 | L46 A44 L47 A43 | A47 L51 A48 L50 | L52 A50 L53 A49 | A55 L59 A56 L58 | L60 A57 L61 A58 | L70 A68 L71 A67 | L72 A70 L73 A69 | L74 A72 L75 A71 | L76 A74 L77 A73
extrude "Extrusão10" cut sketch "Esboço9" against normal blind 2 contours L3 L2 L1 L5
fillet "Arredondamento3" radius 2 5 edges at (21.5, -7, 1) (21.5, 70, 1) (0.5, 70, 1) (89.7, -7, 1) (84.7, -7, 1)
fillet "Arredondamento4" radius 0.5 2 edges at (89.7, 5, 1) (84.7, 5, 1)
sketch "Esboço11" plane through (0, 0, 2) normal (0, 0, 1) x (1, 0, 0)
  line L0 (58.7388, 91) -> (58.7388, 110.4463) projected
  line L1 (109.5, 131) -> (109.5, -5) projected
  line L2 (84.1194, 106.3263) -> (84.1194, 10.4336)
  line L3 (109.5, 63) -> (70.2824, 63)
  line L4 (2.5, 133) -> (107.5, 133) projected
  line L5 (23.5, -7) -> (82.7, -7) projected
  circle A0 centre (84.1194, 107) radius 2.5
  circle A1 centre (84.1194, 19) radius 2.5
  point P0 (0, 0)
  dimension "d100" = 70
  dimension "d101" = 140
  dimension "d102" = 25.3806
  dimension "d103" = 5
  dimension "d104" = 5
  dimension "d105" = 44
  dimension "d106" = 44
  constraints: 4 end point, 2 centre point, 2 point on line, 1 horizontal, 1 midpoint, 1 vertical
  measures "d100" distance between parallel lines of L4 L3
  measures "d101" distance between parallel lines of L5 L4
  measures "d102" distance between parallel lines of L1 L2
  measures "d103" diameter of A0
  measures "d104" diameter of A1
  measures "d105" distance from line of L3 A0.centre
  measures "d106" distance from line of L3 A1.centre
extrude "Extrusão11" cut sketch "Esboço11" against normal blind 2
sketch "Esboço12" plane through (0, 0, 2) normal (0, 0, 1) x (1, 0, 0)
  arc A0 (21.5, -5) -> (23.5, -7) centre (23.5, -5) ccw projected
  line L0 (23.5, -7) -> (0.5, -7)
  line L1 (0.5, -7) -> (0.5, 6)
  line L2 (0.5, 6) -> (23.5, 6)
  line L3 (23.5, 6) -> (23.5, -7)
  line L4 (0.5, 131) -> (0.5, 72) projected
  point P0 (0, 0)
  dimension "d109" = 13
  constraints: 8 end point, 2 parallel, 2 perpendicular
  measures "d109" distance of L0.end L1.end
extrude "Extrusão12" add sketch "Esboço12" against normal blind 2
fillet "Arredondamento5" radius 2 3 edges at (0.5, -7, 1) (0.5, 6, 1) (21.5, 6, 1)
sketch "Esboço13" plane through (0, 0, 2) normal (0, 0, 1) x (1, 0, 0)
  line L0 (21.5, 68) -> (21.5, 8) projected
  arc A0 (19.5, 6) -> (21.5, 8) centre (19.5, 8) ccw projected
  line L1 (19.5, 6) -> (2.5, 6) projected
  arc A1 (21.5, 68) -> (19.5, 70) centre (19.5, 68) ccw projected
  line L2 (2.5, 70) -> (19.5, 70) projected
  line L3 (2.5, 3) -> (19.5, 3)
  arc A2 (19.5, 3) -> (24.5, 8) centre (19.5, 8) ccw
  line L4 (24.5, 8) -> (24.5, 68)
  arc A3 (24.5, 68) -> (19.5, 73) centre (19.5, 68) ccw
  line L5 (19.5, 73) -> (2.5, 73)
  line L6 (2.5, 73) -> (0.5, 73)
  line L7 (0.5, 131) -> (0.5, 72) projected
  line L8 (2.5, 3) -> (0.5, 3)
  arc A4 (2.5, 6) -> (0.5, 4) centre (2.5, 4) ccw projected
  line L9 (0.5, 4) -> (0.5, -5) projected
  arc A5 (0.5, 72) -> (2.5, 70) centre (2.5, 72) ccw projected
  point P0 (0, 0)
  dimension "d113" = 3
  constraints: 10 end point, 4 point on circle, 2 centre point, 2 horizontal, 1 point on line, 4 other
  measures "d113" distance between parallel lines of L0 L4
extrude "Extrusão13" add sketch "Esboço13" along normal blind 23
fillet "Arredondamento6" radius 0.5 14 edges at (23.0355, 71.5355, 25) (10, 73, 25) (23.0355, 4.4645, 25) (10, 3, 25) (24.5, 38, 25) (20.9142, 6.5858, 25) (11, 6, 25) (1.0858, 5.4142, 25) (0.5, 3.5, 25) (20.9142, 69.4142, 25) (11, 70, 25) (1.0858, 70.5858, 25) (0.5, 72.5, 25) (21.5, 38, 25)
fillet "Arredondamento7" radius 1 5 edges at (23.0355, 4.4645, 2) (24.5, 38, 2) (23.0355, 71.5355, 2) (10, 73, 2) (10, 3, 2)
equation "\"d13\" = d12"
equation "\"d16\" = d15"
equation "\"d20\" = d19"
equation "\"d70\" = d18"
equation "\"d103\" = d104"
